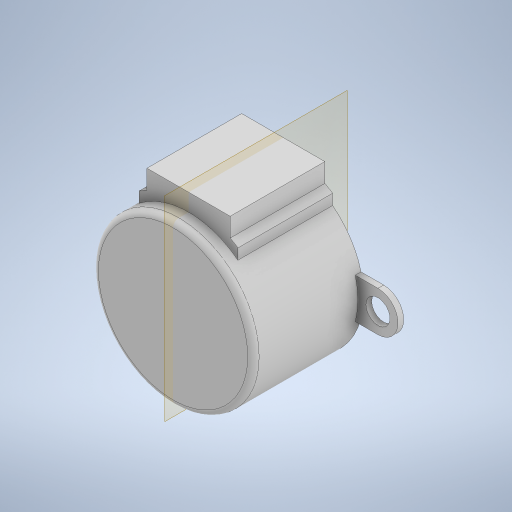
# Autodesk Inventor part: Motor
Saved by Autodesk Inventor 2023 (Build 270158000, 158)
## iProperties
Created: 2023-11-20
Part Number: Motor
Material: Všeobecné
Document SubType Name: Modeling
Designer: M.Ćmiel
Stock Number: Číslo současti
Mass: 12.9927 g
Surface Area: 33.2008 cm^2
Volume: 12.9927 cm^3
Density: 1 g/cm^3
Appearance: Výchozí
LastSaveDate: 2023-11-20
Mass: 0 kg
FileName: NORMA SUCAST
Author: M.Ćmiel
Autodesk Inventor part; units mm, degrees
ref_plane "XZ Plane" through (0, 0, 0) normal (0, 1, 0) x (-1, 0, 0)
ref_plane "XY Plane" through (0, 0, 0) normal (0, 0, 1) x (1, 0, 0)
sketch "Náčrt1" plane through (0, 0, 0) normal (0, 0, 1) x (1, 0, 0)
  line L0 (0, 19.6) -> (0, -19.6) projected
  line L1 (-19.6, 0) -> (19.6, 0) projected
  circle A0 centre (0, 0) radius 14
  dimension "d0" = 28
  constraints: 1 centre point, 1 coincident
  measures "d0" diameter of A0
extrude "Vysunutí1" add sketch "Náčrt1" along normal blind 19.2
fillet "Zaoblení1" radius 1 1 edges at (-14, 0, 19.2)
sketch "Náčrt2" plane through (0, 0, 0) normal (0, 0, -1) x (-1, 0, 0)
  line L0 (-7.25, 11) -> (7.25, 11)
  line L1 (7.25, 11) -> (7.25, 17)
  line L2 (7.25, 17) -> (-7.25, 17)
  line L3 (-7.25, 17) -> (-7.25, 11)
  circle A0 centre (0, 0) radius 14 projected
  line L4 (-7.25, 11) -> (7.25, 17) construction
  line L5 (7.25, 11) -> (-7.25, 17) construction
  circle A1 centre (0, 0) radius 15.5
  line L6 (-8.6, 12.8953) -> (-8.6, 11.0472)
  line L7 (8.6, 12.8953) -> (8.6, 11.0472)
  point P0 (0, 14)
  point P1 (0, 14)
  point P2 (7.25, 13.6999)
  point P3 (-7.25, 13.6999)
  dimension "d4" = 14.5
  dimension "d5" = 31
  dimension "d6" = 17.2
  dimension "d7" = 1.35
  dimension "d8" = 1.35
  dimension "d9" = 1.5
  constraints: 16 end point, 5 point on circle, 3 midpoint, 2 parallel, 2 vertical, 1 centre point, 1 horizontal, 1 perpendicular, 1 vertical alignment
  measures "d4" distance of L1.end L2.end
  measures "d6" distance between parallel lines of L7 L6
  measures "d7" distance between parallel lines of L3 L6
  measures "d8" distance between parallel lines of L1 L7
  measures "d9" radial gap between concentric circles of A0 A1
extrude "Vysunutí2" add sketch "Náčrt2" against normal blind 16.5 contours A0 L6 A1 L3 | L3 A1 L1 A0 | L1 A1 L7 A0 | L3 L2 L1 A1
sketch "Náčrt3" plane through (0, 0, 0) normal (0, 0, -1) x (-1, 0, 0)
  circle A0 centre (0, -8) radius 4.6
  line L0 (0, -12.6) -> (0, -14) construction
  arc A1 (-8.6, 11.0472) -> (8.6, 11.0472) centre (0, 0) ccw construction
  dimension "d12" = 9.2
  dimension "d14" = 1.4
  constraints: 2 end point, 1 point on circle, 1 vertical, 1 vertical alignment, 2 other
  measures "d14" distance of L0.start L0.end
extrude "Vysunutí3" add sketch "Náčrt3" along normal blind 1.7
sketch "Náčrt4" plane through (0, -8, -1.7) normal (0, 0, -1) x (-1, 0, 0)
  circle A0 centre (0, 0) radius 4.6 projected
  circle A1 centre (0, 0) radius 2.5
  line L0 (-1.475, 2.0185) -> (-1.475, -2.0185)
  line L1 (1.475, 2.0185) -> (1.475, -2.0185)
  point P0 (0, 8)
  dimension "d17" = 5
  dimension "d18" = 2.95
  constraints: 4 end point, 4 point on circle, 2 parallel, 1 centre point, 1 coincident, 1 vertical
  measures "d17" diameter of A1
  measures "d18" distance between parallel lines of L0 L1
extrude "Vysunutí4" add sketch "Náčrt4" along normal blind 8 contours L1 A1 L0
sketch "Náčrt5" plane through (0, -8, -1.7) normal (0, 0, -1) x (-1, 0, 0)
  arc A0 (1.475, 2.0185) -> (-1.475, 2.0185) centre (0, 0) ccw projected
  circle A1 centre (0, 0) radius 2.5
  point P0 (0, 8)
  point P1 (-1.475, 2.0185)
  point P2 (1.475, 2.0185)
  constraints: 1 centre point, 1 coincident
extrude "Vysunutí5" add sketch "Náčrt5" along normal blind 2
sketch "Sketch6" plane through (0, 0, 0) normal (0, 0, -1) x (-1, 0, 0)
  line L0 (-17.5, 0) -> (17.5, 0) construction
  line L1 (-17.5, -3.5) -> (17.5, -3.5)
  line L2 (17.5, 3.5) -> (-17.5, 3.5)
  arc A0 (-17.5, 3.5) -> (-17.5, -3.5) centre (-17.5, 0) ccw
  arc A1 (17.5, -3.5) -> (17.5, 3.5) centre (17.5, 0) ccw
  circle A2 centre (-17.5, 0) radius 2.1
  circle A3 centre (17.5, 0) radius 2.1
  point P0 (0, 0)
  dimension "d23" = 4.2
  dimension "d24" = 35
  dimension "d25" = 7
  constraints: 8 end point, 4 centre point, 4 point on circle, 4 tangent, 2 coincident, 1 equal radius, 1 horizontal, 1 midpoint, 1 parallel
  measures "d23" diameter of A2
  measures "d24" distance of L0.end L0.start
  measures "d25" distance between parallel lines of L1 L2
extrude "Extrusion6" add sketch "Sketch6" against normal blind 1
equation "\"d7\" = d8"
